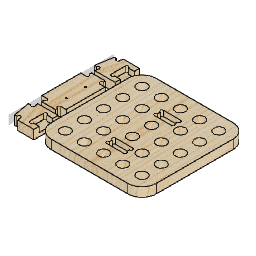
model (Autodesk Fusion 360 design; units mm, degrees)
Autodesk Fusion 360 part; units mm, degrees
sketch "holes" plane through (0, 0, 0) normal (0, 1, 0) x (1, 0, 0) in component "doghome"
  circle A0 centre (28, -28) radius 10
  circle A1 centre (66, -28) radius 10
  circle A2 centre (104, -28) radius 10
  circle A3 centre (142, -28) radius 10
  circle A4 centre (28, -66) radius 10
  circle A5 centre (66, -66) radius 10
  circle A6 centre (104, -66) radius 10
  circle A7 centre (142, -66) radius 10
  circle A8 centre (28, -104) radius 10
  circle A9 centre (66, -104) radius 10
  circle A10 centre (104, -104) radius 10
  circle A11 centre (142, -104) radius 10
  circle A12 centre (28, -142) radius 10
  circle A13 centre (66, -142) radius 10
  circle A14 centre (104, -142) radius 10
  circle A15 centre (142, -142) radius 10
  line L0 (0, 0) -> (208, 0)
  line L1 (208, 0) -> (208, -208)
  line L2 (208, -208) -> (0, -208)
  line L3 (0, -208) -> (0, 0)
  line L4 (28, -28) -> (28, 0) construction
  line L5 (28, -28) -> (0, -28) construction
  circle A16 centre (180, -28) radius 10
  circle A17 centre (180, -66) radius 10
  circle A18 centre (180, -104) radius 10
  circle A19 centre (180, -142) radius 10
  circle A20 centre (28, -180) radius 10
  circle A21 centre (66, -180) radius 10
  circle A22 centre (104, -180) radius 10
  circle A23 centre (142, -180) radius 10
  circle A24 centre (180, -180) radius 10
  arc A25 (0, -180) -> (28, -208) centre (28, -180) ccw
  arc A26 (180, -208) -> (208, -180) centre (180, -180) ccw
  arc A27 (208, -28) -> (180, 0) centre (180, -28) ccw
  arc A28 (28, 0) -> (0, -28) centre (28, -28) ccw
  dimension "d10" = 20
  dimension "d13" = 38
  dimension "d15" = 28
  dimension "d20" = 208
  dimension "d21" = 208
  constraint horizontal L0
  constraint vertical L1
  constraint horizontal L2
  constraint vertical L3
  constraint coincident L0.start L3.end
  constraint coincident A0.centre L4.start
  constraint coincident L0 L4.end
  constraint perpendicular L0 L4
  constraint coincident L3 L5.end
  constraint perpendicular L3 L5
  constraint equal L4 L5
  constraint tangent L2 A25
  constraint coincident L2 A25.end
  constraint coincident L3 A25.start
  constraint tangent L1 A26
  constraint coincident L1 A26.end
  constraint coincident L2 A26.start
  constraint tangent L1 A27
  constraint coincident L1 A27.start
  constraint coincident L0 A27.end
  constraint tangent L0 A28
  constraint tangent L3 A28
  constraint tangent L2 A26
  constraint tangent L3 A25
  constraint tangent L0 A27
  constraint equal A25 A28
  constraint equal A26 A28
  constraint equal A27 A28
  measures "d10" diameter of A0
  measures "d15" distance of A0.centre L4.end
  measures "d20" distance of L0.start L2.end
  measures "d21" distance of L0.start L0.end
sketch "alt holes" plane through (0, 0, 0) normal (0, 1, 0) x (1, 0, 0) in component "doghome"
  circle A0 centre (85, -104) radius 10
  circle A1 centre (123, -104) radius 10
  line L0 (28, -104) -> (85, -104) construction
  line L1 (85, -104) -> (123, -104) construction
  line L2 (123, -104) -> (180, -104) construction
  point P0 (28, -104)
  point P1 (180, -104)
  dimension "d27" = 20
  dimension "d30" = 38
  constraint equal A0 A1
  constraint coincident P0 L0.start
  constraint coincident A0.centre L0.end
  constraint coincident A1.centre L1.end
  constraint horizontal L1
  constraint coincident P1 L2.end
  constraint collinear L0 L1
  constraint equal L0 L2
  measures "d27" diameter of A0
  measures "d30" distance of A0.centre A1.centre
extrude "Extrude1" add sketch "holes" along normal blind 18 contours A9 | A10 | A11 | L0 L1 L2 L3 A25 A26 A27 A28 makes body 1 in component "doghome"
extrude "Extrude2" cut sketch "alt holes" along normal up to surface (18 mm away) bodies 1 in component "doghome"
move_body "Move1" bodies 1 to x (1, 0, 0) y (0, 0.984808, -0.173648) z (0, 0.173648, 0.984808) at (0, 1.0855, 6.1564) in component "doghome"
sketch "board support joinery" plane through (0, 17.7265, -3.1257) normal (0, 0.984808, -0.173648) x (-1, 0, 0) in component "doghome"
  circle A0 centre (-85, 110.2513) radius 10
  circle A1 centre (-123, 110.2513) radius 10
  circle A2 centre (-28, 72.2513) radius 10
  circle A3 centre (-66, 34.2513) radius 10
  circle A4 centre (-28, 148.2513) radius 10
  circle A5 centre (-66, 72.2513) radius 10
  circle A6 centre (-104, 72.2513) radius 10
  circle A7 centre (-28, 34.2513) radius 10
  circle A8 centre (-142, 72.2513) radius 10
  circle A9 centre (-142, 34.2513) radius 10
  circle A10 centre (-180, 148.2513) radius 10
  circle A11 centre (-180, 72.2513) radius 10
  circle A12 centre (-180, 34.2513) radius 10
  circle A13 centre (-104, 148.2513) radius 10
  circle A14 centre (-142, 148.2513) radius 10
  circle A15 centre (-180, 110.2513) radius 10
  circle A16 centre (-66, 148.2513) radius 10
  circle A17 centre (-28, 186.2513) radius 10
  circle A18 centre (-180, 186.2513) radius 10
  circle A19 centre (-142, 186.2513) radius 10
  circle A20 centre (-28, 110.2513) radius 10
  circle A21 centre (-104, 34.2513) radius 10
  circle A22 centre (-104, 186.2513) radius 10
  circle A23 centre (-66, 186.2513) radius 10
  arc A24 (-208, 34.2513) -> (-180, 6.2513) centre (-180, 34.2513) ccw
  line L0 (-180, 6.2513) -> (-28, 6.2513)
  arc A25 (-28, 6.2513) -> (0, 34.2513) centre (-28, 34.2513) ccw
  line L1 (0, 34.2513) -> (0, 186.2513)
  arc A26 (0, 186.2513) -> (-28, 214.2513) centre (-28, 186.2513) ccw
  line L2 (-28, 214.2513) -> (-180, 214.2513)
  arc A27 (-180, 214.2513) -> (-208, 186.2513) centre (-180, 186.2513) ccw
  line L3 (-208, 186.2513) -> (-208, 34.2513)
  line L4 (-160.5, 124.2513) -> (-142.5, 124.2513)
  line L5 (-142.5, 124.2513) -> (-142.5, 90.2513)
  line L6 (-142.5, 90.2513) -> (-160.5, 90.2513)
  line L7 (-160.5, 90.2513) -> (-160.5, 124.2513)
  line L8 (-142.5, 110.2513) -> (-123, 110.2513) construction
  arc A28 (-154.0865, 124.2513) -> (-160.5, 124.2513) centre (-157.2933, 124.2513) ccw
  arc A29 (-142.5, 124.2513) -> (-148.9135, 124.2513) centre (-145.7067, 124.2513) ccw
  arc A30 (-160.5, 90.2513) -> (-154.0865, 90.2513) centre (-157.2933, 90.2513) ccw
  arc A31 (-148.9135, 90.2513) -> (-142.5, 90.2513) centre (-145.7067, 90.2513) ccw
  line L9 (-104, 148.2513) -> (-104, 72.2513) construction
  line L10 (-47.5, 90.2513) -> (-47.5, 124.2513)
  arc A32 (-47.5, 124.2513) -> (-53.9135, 124.2513) centre (-50.7067, 124.2513) ccw
  line L11 (-47.5, 124.2513) -> (-65.5, 124.2513)
  arc A33 (-59.0865, 124.2513) -> (-65.5, 124.2513) centre (-62.2933, 124.2513) ccw
  line L12 (-65.5, 124.2513) -> (-65.5, 90.2513)
  arc A34 (-65.5, 90.2513) -> (-59.0865, 90.2513) centre (-62.2933, 90.2513) ccw
  arc A35 (-53.9135, 90.2513) -> (-47.5, 90.2513) centre (-50.7068, 90.2513) ccw
  line L13 (-65.5, 90.2513) -> (-47.5, 90.2513)
  line L14 (-180, 110.2513) -> (-160.5, 110.2513) construction
  dimension "d38" = 18
  dimension "d56" = 3.2067
  dimension "d58" = 20
  dimension "d82" = 14
  constraint horizontal L4
  constraint vertical L5
  constraint horizontal L6
  constraint vertical L7
  constraint coincident A1.centre L8.end
  constraint horizontal L8
  constraint tangent L7 A28
  constraint coincident L4 A28.start
  constraint tangent L5 A29
  constraint coincident L4 A29.end
  constraint tangent L7 A30
  constraint coincident L6 A30.end
  constraint tangent L5 A31
  constraint coincident L6 A31.start
  constraint coincident A13.centre L9.start
  constraint coincident A6.centre L9.end
  constraint equal A30 A31
  constraint equal A28 A30
  constraint equal A29 A30
  constraint symmetric L4.start L9 L10.end
  constraint symmetric L4.end L9 L11.end
  constraint symmetric L5.end L9 L12.end
  constraint symmetric L6.end L9 L10.start
  constraint symmetric A28.start L9 A32.end
  constraint symmetric A28 L9 A32
  constraint symmetric A29.end L9 A33.start
  constraint symmetric A29 L9 A33
  constraint symmetric A30.end L9 A35.start
  constraint symmetric A30 L9 A35
  constraint symmetric A31.start L9 A34.end
  constraint symmetric A31 L9 A34
  constraint coincident L5 L8.start
  constraint coincident A15.centre L14.start
  constraint coincident L7 L14.end
  constraint perpendicular L7 L14
  constraint equal L8 L14
  measures "d38" distance of L4.start L4.end
  measures "d56" radius of A30
  measures "d58" vertical distance of A15.centre L6.end
  measures "d82" distance of L4 L8.start
sketch "side" plane through (0, 0, 0) normal (1, 0, 0) x (0, 1, 0) in component "doghome"
  line L0 (50.0687, 180.2961) -> (23.6742, 30.6053) construction
  line L1 (50.0687, 180.2961) -> (72.3246, 176.3718) construction
  line L2 (72.3246, 176.3718) -> (72.3246, 30.6053) construction
  line L3 (72.3246, 30.6053) -> (23.6742, 30.6053) construction
  line L4 (36.8715, 105.4507) -> (72.3246, 99.1994) construction
  line L5 (72.3246, 126.3733) -> (54.3246, 126.3733)
  line L6 (54.3246, 126.3733) -> (54.3246, 78.3733)
  line L7 (54.3246, 78.3733) -> (72.3246, 78.3733)
  line L8 (72.3246, 78.3733) -> (72.3246, 126.3733)
  line L9 (41.7336, 133.0253) -> (72.3246, 127.6313) construction
  line L10 (32.0093, 77.8761) -> (72.3246, 70.7674) construction
  line L11 (54.3246, 126.3733) -> (40.5607, 126.3733)
  line L12 (54.3246, 78.3733) -> (32.097, 78.3733)
  line L13 (40.5607, 126.3733) -> (32.097, 78.3733)
  point P0 (50.0687, 180.2961)
  point P1 (23.6742, 30.6053)
  point P2 (54.3246, 102.3733)
  dimension "d33" = 36
  dimension "d34" = 18
  dimension "d35" = 48
  dimension "d36" = 28
  dimension "d37" = 28
  constraint coincident P0 L0.start
  constraint coincident P1 L0.end
  constraint perpendicular L0 L1
  constraint vertical L2
  constraint perpendicular L2 L3
  constraint midpoint L0 L4.start
  constraint coincident L2 L4.end
  constraint perpendicular L0 L4
  constraint horizontal L5
  constraint vertical L6
  constraint horizontal L7
  constraint vertical L8
  constraint coincident L2 L5.start
  constraint midpoint L6 P2
  constraint coincident L4 P2
  constraint coincident L0 L9.start
  constraint coincident L2 L9.end
  constraint perpendicular L0 L9
  constraint coincident L0 L10.start
  constraint coincident L2 L10.end
  constraint perpendicular L0 L10
  constraint coincident L0 L11.end
  constraint perpendicular L6 L11
  constraint coincident L0 L12.end
  constraint perpendicular L6 L12
  measures "d33" distance of L4.start L4.end
  measures "d34" distance of L5.start L5.end
  measures "d35" distance of L5.start L7.end
  measures "d36" distance of L4 L10
  measures "d37" distance of L4 L9
extrude "Extrude5" add sketch "side" along normal up to surface (18 mm away) from surface at 47.5 separate body makes body 2 in component "doghome"
extrude "Extrude6" add sketch "side" along normal up to surface (18 mm away) from surface at 142.5 separate body makes body 3 in component "doghome"
extrude "Extrude7" add sketch "side" along normal up to surface (77 mm away) from surface at 65.5 separate body contours L5 L6 L7 L8 makes body 4 in component "doghome"
extrude "Extrude8" add sketch "board support joinery" against normal blind 10.8 contours L4 L5 L6 L7 | L10 L11 L12 L13 bodies 2 3 4 in component "doghome"
extrude "Extrude9" cut sketch "board support joinery" against normal blind 10.8 contours L4 A28 | L4 L5 L6 L7 | L6 A30 | L4 A29 | L6 A31 | L10 L11 L12 L13 | A35 L13 | A32 L11 | A34 L13 | L11 A33 bodies 1 in component "doghome"
sketch "support board relief" plane through (160.5, 0, 0) normal (1, 0, 0) x (0, 1, 0) in component "doghome"
  line L0 (33.3985, 85.7545) -> (32.097, 78.3733)
  line L1 (32.097, 78.3733) -> (72.3246, 78.3733)
  line L2 (72.3246, 78.3733) -> (72.3246, 126.3733)
  line L3 (72.3246, 126.3733) -> (40.5607, 126.3733)
  line L4 (40.5607, 126.3733) -> (39.3026, 119.238)
  line L5 (39.3026, 119.238) -> (28.6666, 121.1134)
  line L6 (28.6666, 121.1134) -> (22.7626, 87.6299)
  line L7 (22.7626, 87.6299) -> (33.3985, 85.7545)
  arc A0 (32.9865, 120.3517) -> (39.3026, 119.238) centre (36.1445, 119.7949) ccw
  arc A1 (33.3985, 85.7545) -> (27.0825, 86.8682) centre (30.2405, 86.3114) ccw
  line L8 (32.9865, 120.3517) -> (39.3026, 119.238)
  line L9 (27.0825, 86.8682) -> (33.3985, 85.7545)
  dimension "d64" = 3.2067
  constraint tangent L4 A0
  constraint coincident L4.end L5.start
  constraint coincident L5 A0.start
  constraint tangent L0 A1
  constraint coincident L7 A1.end
  constraint coincident L0.start L7.end
  constraint equal A0 A1
  measures "d64" radius of A0
extrude "Extrude10" cut sketch "support board relief" against normal up to surface (113 mm away) contours L7 A1 L9 | L5 A0 L8 bodies 2 3 in component "doghome"
sketch "support mount joinery" plane through (47.5, 0, 0) normal (-1, 0, 0) x (0, -1, 0) in component "doghome"
  arc A0 (-39.3026, 119.238) -> (-32.9865, 120.3517) centre (-36.1445, 119.7949) ccw
  line L0 (-39.3026, 119.238) -> (-40.5607, 126.3733)
  line L1 (-40.5607, 126.3733) -> (-72.3246, 126.3733)
  line L2 (-72.3246, 126.3733) -> (-72.3246, 78.3733)
  line L3 (-72.3246, 78.3733) -> (-32.097, 78.3733)
  line L4 (-32.097, 78.3733) -> (-33.3985, 85.7545)
  arc A1 (-27.0825, 86.8682) -> (-33.3985, 85.7545) centre (-30.2405, 86.3114) ccw
  line L5 (-27.0825, 86.8682) -> (-22.7626, 87.6299)
  line L6 (-22.7626, 87.6299) -> (-28.6666, 121.1134)
  line L7 (-28.6666, 121.1134) -> (-32.9865, 120.3517)
  line L8 (-72.3246, 115.9665) -> (-54.3246, 115.9665)
  line L9 (-54.3246, 115.9665) -> (-54.3246, 88.78)
  line L10 (-54.3246, 88.78) -> (-72.3246, 88.78)
  line L11 (-72.3246, 88.78) -> (-72.3246, 115.9665)
  arc A2 (-54.3246, 115.9665) -> (-60.7381, 115.9665) centre (-57.5313, 115.9665) ccw
  arc A3 (-60.7381, 88.78) -> (-54.3246, 88.78) centre (-57.5313, 88.78) ccw
  line L12 (-63.3246, 115.9665) -> (-63.3246, 126.3733) construction
  line L13 (-63.3246, 88.78) -> (-63.3246, 78.3733) construction
  point P0 (-57.5313, 119.1733)
  dimension "d68" = 18
  dimension "d70" = 3.2067
  dimension "d71" = 7.2
  constraint horizontal L8
  constraint vertical L9
  constraint horizontal L10
  constraint vertical L11
  constraint coincident L2 L8.start
  constraint tangent L9 A2
  constraint coincident L8 A2.end
  constraint tangent L9 A3
  constraint coincident L10 A3.start
  constraint equal A2 A3
  constraint midpoint A2 P0
  constraint midpoint L8 L12.start
  constraint coincident L1 L12.end
  constraint perpendicular L1 L12
  constraint midpoint L10 L13.start
  constraint coincident L3 L13.end
  constraint perpendicular L3 L13
  constraint equal L12 L13
  measures "d68" distance of L8.start L8.end
  measures "d70" radius of A2
  measures "d71" distance of L1 P0
extrude "Extrude11" cut sketch "support mount joinery" along normal blind 10.8 from surface at -18 contours L2 L8 L9 L10 L11 | L8 A2 | L10 A3 bodies 2 in component "doghome"
extrude "Extrude12" cut sketch "support mount joinery" against normal blind 10.8 from surface at -95 contours L2 L8 L9 L10 L11 | L8 A2 | L10 A3 bodies 3 in component "doghome"
sketch "mount support joinery" plane through (0, 72.3246, 0) normal (0, 1, 0) x (-1, 0, 0) in component "doghome"
  line L0 (-142.5, 126.3733) -> (-142.5, 78.3733)
  line L1 (-142.5, 78.3733) -> (-65.5, 78.3733)
  line L2 (-65.5, 78.3733) -> (-65.5, 126.3733)
  line L3 (-65.5, 126.3733) -> (-142.5, 126.3733)
  line L4 (-142.5, 102.3733) -> (-65.5, 102.3733) construction
  line L5 (-153.3, 115.9665) -> (-153.3, 102.3733)
  line L6 (-142.5, 102.3733) -> (-142.5, 115.9665)
  line L7 (-148.9135, 115.9665) -> (-153.3, 115.9665)
  arc A0 (-148.9135, 115.9665) -> (-142.5, 115.9665) centre (-145.7068, 115.9665) ccw
  line L8 (-104, 107.9638) -> (-104, 96.7827) construction
  line L9 (-148.9135, 115.9665) -> (-145.7068, 115.9665) construction
  line L10 (-65.5, 102.3733) -> (-65.5, 115.9665)
  line L11 (-54.7, 115.9665) -> (-54.7, 102.3733)
  line L12 (-59.0865, 115.9665) -> (-54.7, 115.9665)
  arc A1 (-65.5, 115.9665) -> (-59.0865, 115.9665) centre (-62.2932, 115.9665) ccw
  line L13 (-142.5, 102.3733) -> (-142.5, 88.78)
  line L14 (-153.3, 88.78) -> (-153.3, 102.3733)
  line L15 (-148.9135, 88.78) -> (-153.3, 88.78)
  arc A2 (-142.5, 88.78) -> (-148.9135, 88.78) centre (-145.7068, 88.78) ccw
  line L16 (-54.7, 88.78) -> (-54.7, 102.3733)
  line L17 (-65.5, 102.3733) -> (-65.5, 88.78)
  line L18 (-59.0865, 88.78) -> (-54.7, 88.78)
  arc A3 (-59.0865, 88.78) -> (-65.5, 88.78) centre (-62.2932, 88.78) ccw
  point P0 (-153.3, 115.9665)
  dimension "d78" = 3.2067
  constraint midpoint L0 L4.start
  constraint midpoint L2 L4.end
  constraint coincident P0 L5.start
  constraint perpendicular L3 L5
  constraint perpendicular L5 L7
  constraint perpendicular L6 L7
  constraint tangent L6 A0
  constraint vertical L8
  constraint midpoint L4 L8
  constraint coincident A0.centre L9.end
  constraint collinear L7 L9
  constraint symmetric L4.start L8 L4.end
  constraint symmetric P0 L8 L11.start
  constraint symmetric L5.end L8 L11.end
  constraint symmetric L6.end L8 L10.end
  constraint symmetric L7.start L8 L12.start
  constraint symmetric A0 L8 A1
  constraint symmetric L6.start L4 L13.start
  constraint symmetric L4 P0 L14.start
  constraint symmetric L4 L5.end L14.end
  constraint symmetric L4 L6.end L13.end
  constraint symmetric L4 L7.start L15.start
  constraint symmetric L4 A0 A2
  constraint symmetric L4 L10.start L17.start
  constraint symmetric L4 L10.end L17.end
  constraint symmetric L4 L11.end L16.end
  constraint symmetric L4 L11.start L16.start
  constraint symmetric L4 L12.start L18.start
  constraint symmetric L4 A1 A3
  measures "d78" radius of A0
extrude "Extrude13" add sketch "mount support joinery" against normal up to surface (18 mm away) contours L0 L5 L6 L7 A0 L13 L14 L15 A2 | L2 L10 L11 L12 A1 L16 L17 L18 A3 bodies 4 in component "doghome"
sketch "screw holes" plane through (0, 54.3246, 0) normal (0, -1, 0) x (1, 0, 0) in component "doghome"
  line L0 (142.5, 115.9665) -> (142.5, 126.3733)
  line L1 (142.5, 126.3733) -> (65.5, 126.3733)
  line L2 (65.5, 126.3733) -> (65.5, 115.9665)
  arc A0 (59.0865, 115.9665) -> (65.5, 115.9665) centre (62.2932, 115.9665) ccw
  line L3 (59.0865, 115.9665) -> (54.7, 115.9665)
  line L4 (54.7, 115.9665) -> (54.7, 88.78)
  line L5 (54.7, 88.78) -> (59.0865, 88.78)
  arc A1 (65.5, 88.78) -> (59.0865, 88.78) centre (62.2932, 88.78) ccw
  line L6 (65.5, 88.78) -> (65.5, 78.3733)
  line L7 (65.5, 78.3733) -> (142.5, 78.3733)
  line L8 (142.5, 78.3733) -> (142.5, 88.78)
  arc A2 (148.9135, 88.78) -> (142.5, 88.78) centre (145.7068, 88.78) ccw
  line L9 (148.9135, 88.78) -> (153.3, 88.78)
  line L10 (153.3, 88.78) -> (153.3, 115.9665)
  line L11 (153.3, 115.9665) -> (148.9135, 115.9665)
  arc A3 (142.5, 115.9665) -> (148.9135, 115.9665) centre (145.7068, 115.9665) ccw
  line L12 (54.7, 102.3733) -> (87.5667, 102.3733) construction
  line L13 (87.5667, 102.3733) -> (120.4333, 102.3733) construction
  line L14 (120.4333, 102.3733) -> (153.3, 102.3733) construction
  circle A4 centre (85.0667, 107.1233) radius 1.6034
  circle A5 centre (122.9333, 107.1233) radius 1.6034
  line L15 (120.4333, 102.3733) -> (122.9333, 107.1233) construction
  line L16 (122.9333, 107.1233) -> (85.0667, 107.1233) construction
  line L17 (85.0667, 107.1233) -> (87.5667, 102.3733) construction
  line L18 (85.0667, 107.1233) -> (85.0667, 93.7912) construction
  dimension "d83" = 3.2067
  dimension "d86" = 4.75
  dimension "d87" = 2.5
  constraint midpoint L4 L12.start
  constraint perpendicular L4 L12
  constraint perpendicular L4 L13
  constraint midpoint L10 L14.end
  constraint perpendicular L10 L14
  constraint equal L12 L13
  constraint equal L13 L14
  constraint equal A4 A5
  constraint coincident A5.centre L15.end
  constraint coincident A4.centre L16.end
  constraint horizontal L16
  constraint equal L15 L17
  constraint perpendicular L16 L18
  measures "d83" diameter of A4
  measures "d86" distance of L12 A4.centre
  measures "d87" horizontal distance of L12.end A4.centre
extrude "Extrude14" cut sketch "screw holes" against normal blind 2 contours A4 | A5 bodies 4 in component "doghome"
move_body "Move2" bodies 4 to x (1, 0, 0) y (0, 0, -1) z (0, 1, 0) at (0, -6.0487, 70.6978) in component "doghome"
move_body "Move3" bodies 3 to x (0, 0, -1) y (0, 1, 0) z (1, 0, 0) at (82.1267, 50, 158.8733) in component "doghome"
move_body "Move4" bodies 2 to x (0, 0, 1) y (0, 1, 0) z (-1, 0, 0) at (125.8733, 50, -49.1267) in component "doghome"
move_body "Move5" bodies 1 to x (1, 0, 0) y (0, -0.173648, 0.984808) z (0, -0.984808, -0.173648) at (0, 342.3278, -1.6511) in component "doghome"
component "doghome" placed x (1, 0, 0) y (0, 1, 0) z (0, 0, 1) at (0, 0, 0)
component "doghome" placed x (1, 0, 0) y (0, 1, 0) z (0, 0, 1) at (0, 0, 0)
equation "angle = 10 deg"
equation "t = 18 mm"
equation "width = 5"
equation "height = 5"
equation "spacing = 20 mm + t"
equation "d11 = width"
equation "d12 = height"
equation "d13 = spacing"
equation "d14 = -spacing"
equation "d15 = spacing - d10 / 2"
equation "d16 = t"
equation "d20 = 2 * d15 + height * spacing - spacing"
equation "d21 = d15 * 2 + width * spacing - spacing"
equation "d30 = spacing"
equation "d33 = 2 * t"
equation "d34 = t"
equation "d36 = spacing - 10 mm"
equation "d37 = d36"
equation "d38 = t"
equation "bitRad = 1/4\" / 2 * 1.01"
equation "d56 = bitRad"
equation "joineryDepth = t - joineryMargin"
equation "d60 = -joineryDepth"
equation "d62 = -joineryDepth"
equation "d64 = bitRad"
equation "joineryMargin = t * 0.4"
equation "d68 = t"
equation "d70 = bitRad"
equation "d71 = joineryMargin"
equation "d73 = joineryDepth"
equation "d76 = -joineryDepth"
equation "d78 = bitRad"
equation "d83 = bitRad"
named bodies: "board", "support", "support (1)", "mount"
